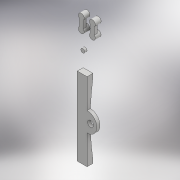
# Autodesk Inventor part: mano
Saved by Autodesk Inventor 2017 (Build 210142000, 142)
## iProperties
Created: 2018-06-27
Part Number: mano
Material: Generic
Document SubType Name: Modeling
Designer: Carolina Lema
Density: 1 g/cm^3
Appearance: Default
Author: Carolina Lema
Autodesk Inventor part; units mm, degrees
ref_plane "YZ Plane" through (0, 0, 0) normal (1, 0, 0) x (0, 1, 0)
ref_plane "XZ Plane" through (0, 0, 0) normal (0, 1, 0) x (-1, 0, 0)
ref_plane "XY Plane" through (0, 0, 0) normal (0, 0, 1) x (1, 0, 0)
sketch "Sketch1" plane through (0, 0, 0) normal (0, 1, 0) x (-1, 0, 0)
  line L0 (0, 0) -> (5, 0)
  line L1 (5, 0) -> (5, -40)
  line L2 (5, -40) -> (0, -40)
  arc A0 (0, -15) -> (0, -25) centre (0, -20) ccw
  line L3 (0, -40) -> (0, -25)
  line L4 (0, -15) -> (0, 0)
  dimension "d0" = 5
  dimension "d1" = 40
  constraints: 10 end point, 3 parallel, 2 point on circle, 1 centre point, 1 horizontal, 1 perpendicular
  measures "d0" distance of L1.end L2.end
  measures "d1" distance of L0.end L1.end
extrude "Extrusion1" add sketch "Sketch1" along normal blind 3
sketch "Sketch2" plane through (-5, 0, -40) normal (-1, 0, 0) x (0, 0, 1)
  line L0 (0, 3) -> (40, 3) projected
  line L1 (40, 3) -> (38, 3)
  line L2 (40, 3) -> (25, 3) projected
  line L3 (15, 3) -> (0, 3) projected
  line L4 (0, 3) -> (2, 3)
  arc A0 (2, 3) -> (38, 3) centre (20, 119.5843) ccw
  point P0 (40, 0)
  dimension "d4" = 2
  dimension "d5" = 2
  constraints: 4 end point, 2 point on circle, 2 point on line, 1 centre point
  measures "d4" distance of L0.end L1.end
  measures "d5" distance of L0.start L4.end
extrude "Extrusion2" cut sketch "Sketch2" against normal blind 10
sketch "Sketch3" plane through (0, 0, 0) normal (0, -1, 0) x (1, 0, 0)
  arc A0 (0, -25) -> (0, -15) centre (0, -20) ccw projected
  circle A1 centre (1.7985, -20) radius 1.5
  point P0 (0, 0)
  dimension "d8" = 3
  constraints: 1 centre point
  measures "d8" diameter of A1
extrude "Extrusion3" cut sketch "Sketch3" against normal blind 10
sketch "Sketch4" plane through (0, 0, 0) normal (0, -1, 0) x (1, 0, 0)
  circle A0 centre (-2.9675, 25.1787) radius 1.5
  circle A1 centre (-2.9675, 19.1787) radius 1.5
  line L0 (-1.9675, 24.0607) -> (-1.9675, 20.2967)
  line L1 (-3.9675, 24.0607) -> (-3.9675, 20.2967)
  circle A2 centre (2.6977, 25.1787) radius 1.5
  circle A3 centre (2.6977, 19.1787) radius 1.5
  line L2 (3.6977, 24.0607) -> (3.6977, 20.2967)
  line L3 (1.6977, 24.0607) -> (1.6977, 20.2967)
  point P0 (0, 0)
  dimension "d11" = 3
  dimension "d14" = 3
  dimension "d17" = 3
  dimension "d18" = 3
  constraints: 8 end point, 8 point on circle, 4 centre point
  measures "d11" diameter of A0
  measures "d14" diameter of A1
  measures "d17" diameter of A2
  measures "d18" diameter of A3
extrude "Extrusion4" add sketch "Sketch4" against normal blind 1.5 contours A0 L0 A1 L1 | A2 L2 A3 L3
sketch "Sketch6" plane through (0, 0, 0) normal (0, -1, 0) x (1, 0, 0)
  circle A0 centre (-2.2031, 10.4312) radius 1
  point P0 (0, 0)
  dimension "d27" = 2
  constraints: 1 centre point
  measures "d27" diameter of A0
extrude "Extrusion6" add sketch "Sketch6" against normal blind 1.2
sketch "Sketch7" plane through (0, 0, 0) normal (0, -1, 0) x (1, 0, 0)
  circle A0 centre (-2.9675, 25.1787) radius 1.5
  circle A1 centre (-2.9675, 19.1787) radius 1.5
  line L0 (-1.9675, 24.0607) -> (-1.9675, 20.2967)
  line L1 (-3.9675, 24.0607) -> (-3.9675, 20.2967)
  circle A2 centre (2.6977, 25.1787) radius 1.5
  circle A3 centre (2.6977, 19.1787) radius 1.5
  line L2 (3.6977, 24.0607) -> (3.6977, 20.2967)
  line L3 (1.6977, 24.0607) -> (1.6977, 20.2967)
  point P0 (0, 0)
  dimension "d30" = 3
  dimension "d31" = 3
  dimension "d32" = 3
  dimension "d33" = 3
  constraints: 8 end point, 8 point on circle, 4 centre point
  measures "d30" diameter of A0
  measures "d31" diameter of A1
  measures "d32" diameter of A2
  measures "d33" diameter of A3
extrude "Extrusion7" add sketch "Sketch7" against normal blind 3 contours A0 | A1 | A2 | A3
body "Solid1"
